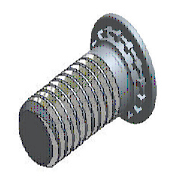
# Autodesk Inventor part: FH4-M5-8
Saved by Autodesk Inventor 2025.2 (Build 292293000, 293)
## iProperties
IsCustomPart: 0
Created: 2024-01-20
Part Number: FH4-M5-8
Material: Stal nierdzewna
Catalog Web Link: www.pemnet.com
Description: PEM Śruba dwustronna samozaciskowa FH4 FHP - Metryczny
Vendor: PennEngineering®
Document SubType Name: Modeling
Standard: PEM
Designer: tadek
Manufacturer: PennEngineering®
Language: pl-PL
Size Designation: FH4-M5-8
Categories: <MemberInstance><Categories><Category DisplayName="Blacha" InternalName="21944ee9-ad4d-44c9-9b1e-873eb7935d2a" Mnemonic="PEM"><Category DisplayName="Śruby dwustronne" InternalName="a2188e1b-484b-4305-8bf4-ec5c89769453" Mnemonic="pemStuds"><CategoryParameter DisplayName="Oznaczenie serii gwintów" InternalName="03190524-7752-4605-8d0f-16dbfc9a5486" Mnemonic="thrserdsgn"/><CategoryParameter DisplayName="Średnica wałka" InternalName="0798fc74-c739-4cf2-a250-69b5137ecf0b" Mnemonic="grpdia"/><CategoryParameter DisplayName="Gwintów na jednostkę" InternalName="18c8b170-0f21-485b-b6b0-effffc919500" Mnemonic="thrperunit1"/><CategoryParameter DisplayName="Długość nominalna" InternalName="2b53957e-0aee-43be-b71a-49b2debece46" Mnemonic="nomlen"/><CategoryParameter DisplayName="Średnica otworu" InternalName="35967fbd-b0ea-4bd0-85e9-351650fbe2ab" Mnemonic="SMBHD"/><CategoryParameter DisplayName="Długość trzonka" InternalName="4f3018fe-66ab-43a1-8110-181b2668c0c7" Mnemonic="shnklen"/><CategoryParameter DisplayName="Oznaczenie gwintu" InternalName="5793e1d1-8c6a-4152-86f4-a921fb5aab9e" Mnemonic="thrdesign"/><CategoryParameter DisplayName="Minimalna grubość blachy" InternalName="5b7d4485-c0aa-4517-a946-c6a5a269b27c" Mnemonic="SMBMIST"/><CategoryParameter DisplayName="Długość gwintu" InternalName="6caf2edf-e86f-4e63-80ff-b45250d5ceee" Mnemonic="thrlen"/><CategoryParameter DisplayName="Klasa gwintu" InternalName="91059bbb-7712-419d-8465-db77f0d91a13" Mnemonic="thrclss"/><CategoryParameter DisplayName="Typ gwintu" InternalName="a3715b49-09e1-4797-90ad-cbfe5ea9b6ea" Mnemonic="thrtype"/><CategoryParameter DisplayName="Długość uchwytu" InternalName="a513e428-3fb5-4a90-abdd-be9a7d5dab44" Mnemonic="grplen"/><CategoryParameter DisplayName="Średnica nominalna" InternalName="ca11677f-f1e9-4208-b7dc-003eed8d1536" Mnemonic="nomdia"/></Category></Category><Category DisplayName="TypDanych" InternalName="23b78d0f-2648-40c6-8793-ca6db495c9e8" Mnemonic="DATATYPE"><CategoryParameter DisplayName="NazwaWyświetlana" InternalName="05415f3d-3907-474b-a020-eb9d644f4cf3" Mnemonic="DISPLAYNAME"/><CategoryParameter DisplayName="Standardowe" InternalName="0c0a119c-1e12-4c84-803f-101930972f5e" Mnemonic="STANDARD"/><CategoryParameter DisplayName="Opis" InternalName="13903e3d-64b1-4950-80da-f627842ea37f" Mnemonic="DESCRIPTION"/><CategoryParameter DisplayName="Oznaczenie" InternalName="2675968c-4ce5-49e0-a4f5-552d29089031" Mnemonic="DESIGNATION"/><CategoryParameter DisplayName="Wiersz domyślny" InternalName="2af9ec52-faaa-4026-b378-f9fa4afca842" Mnemonic="DEFAULTROW"/><CategoryParameter DisplayName="Nazwa folderu" InternalName="3f06958e-8713-4116-9be7-ed6184ecc97b" Mnemonic="FOLDERNAME"/><CategoryParameter DisplayName="Wskazówki do poprawek" InternalName="45a75005-10b1-4dfc-8d6d-dfe629f0b93c" Mnemonic="REVISIONGUID"/><CategoryParameter DisplayName="Nazwa pliku" InternalName="8b46a4cc-9585-4fed-90c3-899f57e09a73" Mnemonic="FILENAME"/><CategoryParameter DisplayName="OrgStd" InternalName="8f5914e1-4693-403f-8ab5-d37768198c9d" Mnemonic="STDSORG"/><CategoryParameter DisplayName="Wersja rodziny" InternalName="914462f6-6e19-4b14-ba84-155b9680b1d0" Mnemonic="FAMILYREVISION"/><CategoryParameter DisplayName="Poprawka standardowa" InternalName="91d5a463-65c2-4fde-b823-3b7fea5e8e17" Mnemonic="STANDARDREVISION"/><CategoryParameter DisplayName="Zmiana elementu" InternalName="a65d44b9-392f-4f4f-857b-e4b3d54996fe" Mnemonic="MEMBERREVISION"/><CategoryParameter DisplayName="FormatKlipu" InternalName="bc51e27b-3422-4e78-93ef-cec197ddf230" Mnemonic="CLIPFORMAT"/><CategoryParameter DisplayName="Producent" InternalName="cd6c7a72-a28a-4e50-99a9-2c7f4e13e5ad" Mnemonic="MANUFACTURER"/><CategoryParameter DisplayName="NazwaWewnętrzna" InternalName="cf1d0246-76d9-4b4a-8305-fa0409afb5c1" Mnemonic="INTERNALNAME"/><CategoryParameter DisplayName="CzyMetryczne" InternalName="e2385c5b-1ea4-4823-96a8-8de651266ec3" Mnemonic="ISMETRIC"/><Category DisplayName="Część" InternalName="c0e0b642-3bcb-4cc8-9e80-f96d35c4afa4" Mnemonic="PART"><CategoryParameter DisplayName="Numer części" InternalName="016b6077-bfbe-49bd-92c9-d8d59c39c941" Mnemonic="PARTNUMBER"/><CategoryParameter DisplayName="Numer katalogowy" InternalName="4dba7c1c-e26c-444e-836c-b08b433409a8" Mnemonic="STOCKNUMBER"/><CategoryParameter DisplayName="Klucz - materiał" InternalName="5c9a8adb-dd2b-4535-b97f-0a94a95fe41f" Mnemonic="MATERIALKEY"/><CategoryParameter DisplayName="Materiał" InternalName="818a152a-d3c3-49ca-80ee-df7d91421b8e" Mnemonic="MATERIAL"/></Category></Category></Categories><FamilyTemplate Id="PEM Self-Clinching Studs FH4,FHP - Metric"><FamilyTemplateParameters><FamilyTemplateParameter ObjectType="kUserParameterObject" ValueType="xs:double" Id="1" ObjectReferenceKey="CH"/><FamilyTemplateParameter ObjectType="kUserParameterObject" ValueType="xs:double" Id="2" ObjectReferenceKey="D_"/><FamilyTemplateParameter ObjectType="kUserParameterObject" ValueType="xs:double" Id="3" ObjectReferenceKey="H_"/><FamilyTemplateParameter ObjectType="kUserParameterObject" ValueType="xs:double" Id="4" ObjectReferenceKey="H_Size"/><FamilyTemplateParameter ObjectType="kUserParameterObject" ValueType="xs:double" Id="5" ObjectReferenceKey="Length_Code"/><FamilyTemplateParameter ObjectType="kUserParameterObject" ValueType="xs:double" Id="7" ObjectReferenceKey="Max_Hole"/><FamilyTemplateParameter ObjectType="kUserParameterObject" ValueType="xs:double" Id="8" ObjectReferenceKey="Min_Dist"/><FamilyTemplateParameter ObjectType="kUserParameterObject" ValueType="xs:double" Id="9" ObjectReferenceKey="Min_Thick"/><FamilyTemplateParameter ObjectType="kUserParameterObject" ValueType="xs:double" Id="11" ObjectReferenceKey="R_"/><FamilyTemplateParameter ObjectType="kUserParameterObject" ValueType="xs:double" Id="12" ObjectReferenceKey="S_"/><FamilyTemplateParameter ObjectType="kUserParameterObject" ValueType="xs:double" Id="17" ObjectReferenceKey="th_"/><FamilyTemplateParameter ObjectType="kPropertyObject" ValueType="xs:string" Id="100" ObjectReferenceKey="{32853F0F-3444-11d1-9E93-0060B03C1CA6}" SubObjectId="52"/><FamilyTemplateParameter ObjectType="kPropertyObject" ValueType="xs:string" Id="105" ObjectReferenceKey="{32853F0F-3444-11d1-9E93-0060B03C1CA6}" SubObjectId="5"/><FamilyTemplateParameter ObjectType="kPartComponentDefinitionObject" ValueType="xs:string" Id="110" SubObjectId="Material"/><FamilyTemplateParameter ObjectType="kThreadFeatureObject" ValueType="xs:structure" Id="300" ObjectReferenceKey="1002000010000000032d0000000000008000000000000000" SubObjectId="ThreadInfo"><FamilyTemplateParameter ObjectType="" ValueType="xs:string" Id="301" SubObjectId="ThreadClass"/><FamilyTemplateParameter ObjectType="" ValueType="xs:string" Id="302" SubObjectId="ThreadDesignation"/><FamilyTemplateParameter ObjectType="" ValueType="xs:string" Id="303" SubObjectId="ThreadType"/><FamilyTemplateParameter ObjectType="" ValueType="xs:string" Id="304" SubObjectId="Pitch"/></FamilyTemplateParameter></FamilyTemplateParameters></FamilyTemplate><CategoryParameterMap><ParamToTemplateMap><ParamToTemplate CategoryParameter="//CategoryParameter[@InternalName='05415f3d-3907-474b-a020-eb9d644f4cf3']" ConstantValue="PEM Self-Clinching Studs FH4,FHP - Metric"/><ParamToTemplate CategoryParameter="//CategoryParameter[@InternalName='0c0a119c-1e12-4c84-803f-101930972f5e']" ConstantValue="PEM"/><ParamToTemplate CategoryParameter="//CategoryParameter[@InternalName='13903e3d-64b1-4950-80da-f627842ea37f']" ConstantValue="PEM Self-Clinching Studs FH4 FHP - Metric"/><ParamToTemplate CategoryParameter="//CategoryParameter[@InternalName='2af9ec52-faaa-4026-b378-f9fa4afca842']" ConstantValue="1"/><ParamToTemplate CategoryParameter="//CategoryParameter[@InternalName='3f06958e-8713-4116-9be7-ed6184ecc97b']" ConstantValue="PEM Self-Clinching Studs FH4,FHP - Metric"/><ParamToTemplate CategoryParameter="//CategoryParameter[@InternalName='45a75005-10b1-4dfc-8d6d-dfe629f0b93c']" ConstantValue="a4f1bebf-a231-4516-be27-821e2d791a0a"/><ParamToTemplate CategoryParameter="//CategoryParameter[@InternalName='8f5914e1-4693-403f-8ab5-d37768198c9d']" TemplateParameter="101"/><ParamToTemplate CategoryParameter="//CategoryParameter[@InternalName='914462f6-6e19-4b14-ba84-155b9680b1d0']" ConstantValue="11"/><ParamToTemplate CategoryParameter="//CategoryParameter[@InternalName='91d5a463-65c2-4fde-b823-3b7fea5e8e17']" TemplateParameter="103"/><ParamToTemplate CategoryParameter="//CategoryParameter[@InternalName='bc51e27b-3422-4e78-93ef-cec197ddf230']" ConstantValue="CF_INVENTOR.STDPARTS"/><ParamToTemplate CategoryParameter="//CategoryParameter[@InternalName='cd6c7a72-a28a-4e50-99a9-2c7f4e13e5ad']" ConstantValue="PennEngineering®"/><ParamToTemplate CategoryParameter="//CategoryParameter[@InternalName='cf1d0246-76d9-4b4a-8305-fa0409afb5c1']" ConstantValue="ae9463b5-ef13-4067-be61-c2d931d05407"/><ParamToTemplate CategoryParameter="//CategoryParameter[@InternalName='e2385c5b-1ea4-4823-96a8-8de651266ec3']" ConstantValue="true"/><ParamToTemplate CategoryParameter="//CategoryParameter[@InternalName='8b46a4cc-9585-4fed-90c3-899f57e09a73']" ConstantValue="FH4-M5-8"/><ParamToTemplate CategoryParameter="//CategoryParameter[@InternalName='a65d44b9-392f-4f4f-857b-e4b3d54996fe']" ConstantValue="849abe67-8b22-44ae-be36-18f3bdfbfcce"/><ParamToTemplate CategoryParameter="//CategoryParameter[@InternalName='2675968c-4ce5-49e0-a4f5-552d29089031']" TemplateParameter="100"/><ParamToTemplate CategoryParameter="//CategoryParameter[@InternalName='ca11677f-f1e9-4208-b7dc-003eed8d1536']" TemplateParameter="2"/><ParamToTemplate CategoryParameter="//CategoryParameter[@InternalName='35967fbd-b0ea-4bd0-85e9-351650fbe2ab']" TemplateParameter="4"/><ParamToTemplate CategoryParameter="//CategoryParameter[@InternalName='2b53957e-0aee-43be-b71a-49b2debece46']" TemplateParameter="5"/><ParamToTemplate CategoryParameter="//CategoryParameter[@InternalName='6caf2edf-e86f-4e63-80ff-b45250d5ceee']" TemplateParameter="5"/><ParamToTemplate CategoryParameter="//CategoryParameter[@InternalName='818a152a-d3c3-49ca-80ee-df7d91421b8e']" TemplateParameter="110"/><ParamToTemplate CategoryParameter="//CategoryParameter[@InternalName='5b7d4485-c0aa-4517-a946-c6a5a269b27c']" TemplateParameter="9"/><ParamToTemplate CategoryParameter="//CategoryParameter[@InternalName='016b6077-bfbe-49bd-92c9-d8d59c39c941']" TemplateParameter="105"/><ParamToTemplate CategoryParameter="//CategoryParameter[@InternalName='4f3018fe-66ab-43a1-8110-181b2668c0c7']" TemplateParameter="12"/><ParamToTemplate CategoryParameter="//CategoryParameter[@InternalName='a513e428-3fb5-4a90-abdd-be9a7d5dab44']" TemplateParameter="12"/><ParamToTemplate CategoryParameter="//CategoryParameter[@InternalName='91059bbb-7712-419d-8465-db77f0d91a13']" TemplateParameter="301"/><ParamToTemplate CategoryParameter="//CategoryParameter[@InternalName='5793e1d1-8c6a-4152-86f4-a921fb5aab9e']" TemplateParameter="302"/><ParamToTemplate CategoryParameter="//CategoryParameter[@InternalName='a3715b49-09e1-4797-90ad-cbfe5ea9b6ea']" TemplateParameter="303"/></ParamToTemplateMap></CategoryParameterMap></MemberInstance>
Density: 8 g/cm^3
Appearance: Częściowo polerowany
Author: tadek
Autodesk Inventor part; units mm, degrees
ref_plane "YZ Plane" through (0, 0, 0) normal (1, 0, 0) x (0, 1, 0)
ref_plane "XZ Plane" through (0, 0, 0) normal (0, 1, 0) x (-1, 0, 0)
sketch "Sketch1" plane through (0, 0, 0) normal (0, 1, 0) x (-1, 0, 0)
  line L0 (0, 0) -> (3.1, 0)
  line L1 (3.25, 0.15) -> (3.25, 0.3)
  line L2 (3.1, 0.45) -> (2.75, 0.45)
  line L3 (2.5, 8) -> (0, 8)
  line L4 (0, 8) -> (0, 0)
  line L5 (2.65, 0.675) -> (2.75, 0.675)
  line L6 (2.75, 0.675) -> (2.75, 0.45)
  arc A0 (2.515, 2.0357) -> (2.65, 1.2632) centre (2.8, 1.6875) ccw
  line L7 (2.65, 1.2632) -> (2.65, 0.675)
  arc A1 (3.25, 0.3) -> (3.1, 0.45) centre (3.1, 0.3) ccw
  arc A2 (3.1, 0) -> (3.25, 0.15) centre (3.1, 0.15) ccw
  line L8 (2.5, 2.7) -> (2.5, 8)
  line L9 (2.5, 2.7) -> (1.275, 2.7) construction
  line L10 (2.515, 2.685) -> (2.515, 2.0357)
  line L11 (2.5, 2.7) -> (2.515, 2.685)
  dimension "d0" = 8
  dimension "d1" = 6.5
  dimension "d3" = 0.45
  dimension "d4" = 0.225
  dimension "d7" = 5.3
  dimension "d8" = 0.45
  dimension "d9" = 5.5
  dimension "d11" = 0.15
  dimension "d35" = 1.0125
  dimension "d41" = 5
  dimension "d43" = 2.7
  dimension "d44" = 5.03
  dimension "d45" = 45
  dimension "d49" = 0.15
  constraints: 24 end point, 6 point on circle, 5 parallel, 5 perpendicular, 4 tangent, 3 centre point, 1 equal radius, 1 horizontal
  measures "d0" distance between parallel lines of L3 L0
  measures "d1" diameter of L1 L4
  measures "d3" distance between parallel lines of L2 L0
  measures "d4" distance between parallel lines of L5 L2
  measures "d7" diameter of L7 L4
  measures "d8" radius of A0
  measures "d9" diameter of L6 L4
  measures "d11" radius of A1
  measures "d35" distance from line of A0.centre L5
  measures "d41" diameter of L8 L4
  measures "d43" distance between parallel lines of L9 L0
  measures "d44" diameter of L10 L4
  measures "d45" angle of L11 L9
  measures "d49" distance from line of L7 A0.centre
revolve "Obrót1" add sketch "Sketch1" angle 360 about axis through (0, 0, 8) along (0, 0, -1)
thread "Gwint1" size "M5x0.8" class "6g" standard "ANSI Metric M Profile" length 5.3
chamfer "Faza1" distance 0.3 angle 45 1 edges at (2.5, 0, 8)
ref_plane "Work Plane1" through (0, 0, 0.9) normal (0, 0, 1) x (1, 0, 0)
sketch "Sketch2" plane through (0, 0, 0.9) normal (0, 0, 1) x (1, 0, 0)
  line L0 (0, 0) -> (0, 2.3973) construction
  circle A0 centre (0, 0) radius 2.875
  line L1 (-0.2, 2.6424) -> (-0.2, 2.868)
  line L2 (0.2, 2.6424) -> (0.2, 2.868)
  circle A1 centre (0, 0) radius 2.65 projected
  dimension "d27" = 5.75
  dimension "d29" = 0.4
  constraints: 6 end point, 4 point on circle, 2 parallel, 1 centre point, 1 coincident, 1 vertical, 1 other
  measures "d27" diameter of A0
  measures "d29" distance between parallel lines of L2 L1
extrude "Wyciągnięcie1" add sketch "Sketch2" against normal up to surface (0.45 mm away) draft 3 contours L2 A1 L1 A0 picked at (0.1556, 2.7199)
pattern_circular "Szyk kołowy1" count 13 over 360 about axis through (0, 0, -10) along (0, 0, 1) of "Wyciągnięcie1"
equation "\"d27\" = 0.5 * D_ + 0.5 * H_"
equation "\"d29\" = th_"
equation "\"d16\" = Length_Code - S_"
equation "\"d18\" = CH"
equation "\"d0\" = Length_Code"
equation "\"d1\" = H_"
equation "\"d3\" = 0.166667 * S_"
equation "\"d4\" = 0.0833333 * S_"
equation "\"d7\" = D_ + 2 * R_"
equation "\"d8\" = 3 * R_"
equation "\"d9\" = 0.666667 * D_ + 0.333333 * H_"
equation "\"d11\" = R_"
equation "\"d35\" = 0.375 * S_"
equation "\"d41\" = D_"
equation "\"d43\" = S_"
equation "\"d44\" = D_ + 0.2 * R_"
equation "\"d49\" = R_"
equation "\"Length_Code\" = 8"
equation "\"H_\" = 6.5"
equation "\"S_\" = 2.7"
equation "\"D_\" = 5"
equation "\"d2\" = D_"
equation "\"CH\" = 0.3"
equation "\"R_\" = 0.15"
equation "\"d26\" = 0.333333 * S_"
equation "\"th_\" = 0.4"
equation "\"d36\" = R_"
equation "\"D1\" = 3.1"
equation "\"Max_Hole\" = 5.6"
equation "\"Min_Dist\" = 7.2"
equation "\"H_Size\" = 5"
equation "\"Min_Thick\" = 1"
body "Solid1"
